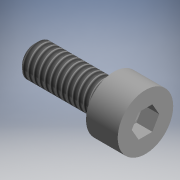
# Autodesk Inventor part: CB4-10_1
Saved by Autodesk Inventor 2017.3 (Build 213256000, 256)
## iProperties
Part Number: CB4-10_1
Material: Generic
Catalog Web Link: www.cadenas.de
Description: CB_1-Hexagon Socket Head Cap Screws
Vendor: MISUMI
Document SubType Name: Modeling
Designer: partserver
Manufacturer: MISUMI
Mass: 0.26199 g
Surface Area: 3.0823 cm^2
Volume: 0.26199 cm^3
Density: 1 g/cm^3
Appearance: PSOLRGB-192-192-192
Category: PARTsolutions
Company: MISUMI
Title: CB4-10_1
Author: Cadenas PARTsolutions
Comments: Hexagon Socket Head Cap Screws
PSOL_IDENT_0: {$CADENAS_DATA\23d-libs\misumi\metric\27_screws_nuts\cb.prj},156 {VTYP=3D},{NB=CB4-10_1},{LINA=CB4-1
PSOL_IDENT_1: 0_1},{NN=CB_1},{DATE=30.03.2018 02:51:37},{GEOMDATE=17.02.2014 00:00:00},{VERSION=},{LINEID=50},{WBV
PSOL_IDENT_2: AR=L},{WBNUMERIC=L}  {NB=CB4-10_1},{LINA=CB4-10_1},{KT=DUMMY},{PN=CB4-10},{MAT=4137 Steel},{HARD=38~
PSOL_IDENT_3: 43HRC},{ST=Black Oxide (Fe3O4)},{M=4},{L=10},{LL=Full Thread},{L1=20},{TYPE=CB},{M1=4.000},{L0=5,6,8
PSOL_IDENT_4: ,10,12,14,15,16,18,20,22,25,30,35,40,45,50,55,60,65,70,75},{NDM=4},{KDM=3.139931},{MP=4x0.7},{P=0.7}
PSOL_IDENT_5: ,{A=7.0},{E=4.0},{B=3.0}
NB: CB4-10_1
NN: CB_1
NT: Hexagon Socket Head Cap Screws
NBSYN: $PN._1
LINA: CB4-10_1
CATALOG: Misumi
PN: CB4-10
MAT: 4137 Steel
HARD: 38~43HRC
ST: Black Oxide (Fe3O4)
M: 4
L: 10
LL: Full Thread
MP: 4x0.7
A: 7
E: 4
B: 3
SUPPLIER: MISUMI
ARTICLENO: CB4-10_1
BOMINFO: CB4-10_1
CREATOR: CADENAS GmbH
Autodesk Inventor part; units mm, degrees
sketch "Sketch_1" plane through (0, 0, 0) normal (0, 0, 1) x (1, 0, 0)
  line L0 (10, 0) -> (-4, 0)
  line L1 (-4, 0) -> (-4, 3.5)
  line L2 (-4, 3.5) -> (0, 3.5)
  line L3 (0, 3.5) -> (0, 2)
  line L4 (0, 2) -> (9.5705, 2)
  line L5 (9.5705, 2) -> (10, 1.5705)
  line L6 (10, 1.5705) -> (10, 0)
  line L7 (10, 0) -> (-4, 0)
  constraints: 16 end point
revolve "Revolution1" add sketch "Sketch_1" angle 360 about axis through (10, 0, 0) along (1, 0, 0)
thread "Thread1" size "M4x0.7" class "6g" standard "ISO Metric profile" length 8.5705
sketch "Sketch2" plane through (-4, 0, 0) normal (-1, 0, 0) x (0, 0, 1)
  point P0 (0, 0)
hole "Hole1" at (-4, 0, 0) direction (1, 0, 0) diameter 3 depth 2 tip angle 150
sketch "Sketch_3" plane through (-4, 0, 0) normal (1, 0, 0) x (0, 0, -1)
  line L0 (-1.5, -0.866) -> (0, -1.7321)
  line L1 (0, -1.7321) -> (1.5, -0.866)
  line L2 (1.5, -0.866) -> (1.5, 0.866)
  line L3 (1.5, 0.866) -> (0, 1.7321)
  line L4 (0, 1.7321) -> (-1.5, 0.866)
  line L5 (-1.5, 0.866) -> (-1.5, -0.866)
  constraints: 12 end point
extrude "Extrusion1" cut sketch "Sketch_3" along normal blind 2
ref_plane "bolt_to_nut_XY" through (10, 0, 0) normal (1, 0, 0) x (0, 0, -1)
ref_plane "bolt_to_nut_YZ" through (10, 0, 0) normal (0, 0, -1) x (0, 1, 0)
ref_plane "bolt_to_nut_ZX" through (10, 0, 0) normal (0, 1, 0) x (1, 0, 0)
ref_plane "screw1_XY" through (0, 0, 0) normal (1, 0, 0) x (0, 0, -1)
ref_plane "screw1_YZ" through (0, 0, 0) normal (0, 0, -1) x (0, 1, 0)
ref_plane "screw1_ZX" through (0, 0, 0) normal (0, 1, 0) x (1, 0, 0)
body "Solid1"
